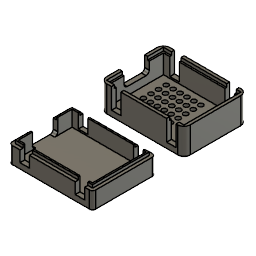
Camera_cover (Autodesk Fusion 360 design; units mm, degrees)
part number: 2026-01-28-19-58-32-867
Autodesk Fusion 360 part; units mm, degrees
note: some values were not read from the file. Chosen so that the rebuilt part matches the saved one: which bodies a step acts on. Set by a fixed rule: which sketch regions a step uses.
sketch "Esquisse1" plane through (0, 0, 0) normal (0, 1, 0) x (1, 0, 0)
  line L0 (23.5, 17) -> (-23.5, 17)
  line L1 (-23.5, 17) -> (-23.5, -17)
  line L2 (-23.5, -17) -> (23.5, -17)
  line L3 (23.5, -17) -> (23.5, 17)
  line L4 (23.5, 17) -> (-23.5, -17) construction
  line L5 (-23.5, 17) -> (23.5, -17) construction
  line L6 (26.5, 20) -> (-26.5, 20)
  line L7 (-26.5, 20) -> (-26.5, -20)
  line L8 (-26.5, -20) -> (26.5, -20)
  line L9 (26.5, -20) -> (26.5, 20)
  line L10 (26.5, 20) -> (-26.5, -20) construction
  line L11 (-26.5, 20) -> (26.5, -20) construction
  dimension "d1" = 47
  dimension "d2" = 34
  dimension "d3" = 40
  dimension "d4" = 53
  constraint horizontal L0
  constraint perpendicular L0 L1
  constraint parallel L0 L2
  constraint parallel L1 L3
  constraint coincident L4 origin
  constraint coincident L5 origin
  constraint horizontal L6
  constraint perpendicular L6 L7
  constraint parallel L6 L8
  constraint parallel L7 L9
  constraint coincident L10 origin
  constraint coincident L11 origin
  measures "d1" distance of L0.start L0.end
  measures "d2" distance of L0.start L2.end
  measures "d3" distance of L6.start L8.end
  measures "d4" distance of L7.end L8.end
extrude "Extrusion1" add sketch "Esquisse1" along normal blind 29 makes body 1
sketch "Esquisse2" plane through (0, 0, 20) normal (0, 0, 1) x (1, 0, 0)
  line L0 (-26.5, 0) -> (26.5, 0)
  line L1 (26.5, 0) -> (26.5, 29)
  line L2 (26.5, 29) -> (-26.5, 29)
  line L3 (-26.5, 29) -> (-26.5, 0)
  line L4 (-26.5, 18) -> (26.5, 18)
  line L5 (26.5, 18) -> (26.5, 17)
  line L6 (26.5, 17) -> (-26.5, 17)
  line L7 (-26.5, 17) -> (-26.5, 18)
  dimension "d8" = 53
  dimension "d9" = 1
  dimension "d10" = 11
  constraint horizontal L4
  constraint vertical L5
  constraint horizontal L6
  constraint vertical L7
  constraint coincident L3 L4.start
  measures "d8" distance of L4.start L4.end
  measures "d9" distance of L4.end L5.end
  measures "d10" distance of L2 L4
extrude "Extrusion2" add sketch "Esquisse1" along normal blind 3 contours L0 L1 L2 L3 bodies 1
extrude "Extrusion3" add sketch "Esquisse1" along normal blind 3 from surface at 26 contours L0 L1 L2 L3 bodies 1
extrude "Extrusion4" cut sketch "Esquisse2" against normal blind 45 contours L1 L3 L4 L5 L6 L7 bodies 1 makes body 2 at (-8.8333, 29, 6.6667)
sketch "Esquisse3" plane through (0, 17, 0) normal (0, 1, 0) x (-1, 0, 0)
  line L0 (-26.5, -20) -> (26.5, -20)
  line L1 (26.5, -20) -> (26.5, 20)
  line L2 (26.5, 20) -> (-26.5, 20)
  line L3 (23.5, -17) -> (-23.5, -17)
  line L4 (-23.5, 17) -> (23.5, 17)
  line L5 (23.5, 17) -> (23.5, -17)
  line L6 (-24.6, -18.1) -> (24.6, -18.1)
  line L7 (24.6, -18.1) -> (24.6, 18.1)
  line L8 (24.6, 18.1) -> (-24.6, 18.1)
  line L9 (-24.6, 18.1) -> (-24.6, -18.1)
  line L10 (-24.6, -18.1) -> (24.6, 18.1) construction
  line L11 (24.6, -18.1) -> (-24.6, 18.1) construction
  line L12 (-26.5, 20) -> (-26.5, -20)
  line L13 (-23.5, -17) -> (-23.5, 17)
  dimension "d18" = 1.1
  dimension "d19" = 1.1
  constraint horizontal L6
  constraint perpendicular L6 L7
  constraint parallel L6 L8
  constraint parallel L7 L9
  constraint coincident L10 origin
  constraint coincident L11 origin
  measures "d18" distance of L3 L6
  measures "d19" distance of L5 L7
extrude "Extrusion5" cut sketch "Esquisse3" against normal blind 2 contours L6 L7 L8 L9 bodies 1
sketch "Esquisse4" plane through (0, 18, 0) normal (0, -1, 0) x (1, 0, 0)
  line L0 (-26.5, -20) -> (26.5, -20)
  line L1 (26.5, 20) -> (-26.5, 20)
  line L2 (-26.5, 20) -> (-26.5, -20)
  line L3 (23.5, -17) -> (-23.5, -17)
  line L4 (-23.5, -17) -> (-23.5, 17)
  line L5 (-23.5, 17) -> (23.5, 17)
  line L6 (21.9, 15.4) -> (-21.9, -15.4) construction
  line L7 (-21.9, 15.4) -> (21.9, -15.4) construction
  line L8 (-24.5, 18) -> (24.5, 18)
  line L9 (24.5, 18) -> (24.5, -18)
  line L10 (24.5, -18) -> (-24.5, -18)
  line L11 (-24.5, -18) -> (-24.5, 18)
  line L12 (-24.5, 18) -> (24.5, -18) construction
  line L13 (24.5, 18) -> (-24.5, -18) construction
  line L14 (26.5, -20) -> (26.5, 20)
  line L15 (23.5, 17) -> (23.5, -17)
  dimension "d51" = 1
  dimension "d74" = 1
  constraint coincident L6 origin
  constraint coincident L7 origin
  constraint horizontal L8
  constraint perpendicular L8 L9
  constraint parallel L8 L10
  constraint parallel L9 L11
  constraint coincident L12 origin
  constraint coincident L13 origin
  measures "d51" distance of L5 L8
  measures "d74" distance of L9 L15
extrude "Extrusion6" add sketch "Esquisse4" along normal blind 1.9 contours L8 L9 L10 L11 bodies 2
fillet "Congé1" radius 2 4 edges at (26.5, 23.5, -20) (26.5, 23.5, 20) (-26.5, 23.5, 20) (-26.5, 23.5, -20) on bodies 2
fillet "Congé2" radius 4 2 edges at (-26.5, 8.5, -20) (-26.5, 8.5, 20) on bodies 1
fillet "Congé2" radius 4 2 edges at (26.5, 8.5, -20) (26.5, 8.5, 20) on bodies 1
sketch "Esquisse5" plane through (0, 0, 20) normal (0, 0, 1) x (1, 0, 0)
  line L0 (-24.5, 29) -> (-24.5, 18)
  line L1 (-24.5, 18) -> (24.5, 18)
  line L2 (24.5, 18) -> (24.5, 29)
  line L3 (24.5, 29) -> (-24.5, 29)
  line L4 (-19.5, 4) -> (-13.5, 4)
  line L5 (-13.5, 4) -> (-13.5, 25)
  line L6 (-13.5, 25) -> (-19.5, 25)
  line L7 (-19.5, 25) -> (-19.5, 4)
  line L8 (-22.5, 0) -> (-22.5, 17)
  line L9 (-22.5, 0) -> (22.5, 0)
  line L10 (21.5, 4) -> (15.5, 4)
  line L11 (15.5, 4) -> (15.5, 25)
  line L12 (15.5, 25) -> (21.5, 25)
  line L13 (21.5, 25) -> (21.5, 4)
  dimension "d30" = 3
  dimension "d31" = 4
  dimension "d32" = 4
  dimension "d34" = 4
  dimension "d35" = 4
  dimension "d71" = 3
  dimension "d72" = 6
  dimension "d73" = 6
  constraint horizontal L4
  constraint vertical L5
  constraint horizontal L6
  constraint vertical L7
  constraint horizontal L10
  constraint vertical L11
  constraint horizontal L12
  constraint vertical L13
  measures "d30" distance of L7 L8
  measures "d31" distance of L4 L9
  measures "d32" distance of L3 L6
  measures "d34" distance of L9 L10
  measures "d35" distance of L3 L12
  measures "d71" distance of L2 L13
  measures "d72" distance of L11 L13
  measures "d73" distance of L5 L7
extrude "Extrusion7" cut sketch "Esquisse5" against normal blind 94 contours L1 L5 L6 L7 | L1 L4 L5 L7 | L1 L10 L11 L13 | L1 L11 L12 L13 bodies 1 2
sketch "Esquisse6" plane through (0, 0, 0) normal (0, -1, 0) x (1, 0, 0)
  line L0 (26.5, -16) -> (26.5, 16)
  line L1 (22.5, 20) -> (-22.5, 20)
  arc A0 (-22.5, 20) -> (-26.5, 16) centre (-22.5, 16) ccw
  line L2 (-26.5, 16) -> (-26.5, -16)
  arc A1 (-26.5, -16) -> (-22.5, -20) centre (-22.5, -16) ccw
  line L3 (-22.5, -20) -> (22.5, -20)
  circle A2 centre (17, 3) radius 4.5
  arc A3 (26.5, 16) -> (22.5, 20) centre (22.5, 16) ccw
  arc A4 (22.5, -20) -> (26.5, -16) centre (22.5, -16) ccw
  dimension "d38" = 9
  dimension "d39" = 17
  dimension "d41" = 9.5
  measures "d38" diameter of A2
  measures "d39" distance of L1 A2.centre
  measures "d41" distance of L0 A2.centre
hole "Perçage1" at (5.0138, 0, -12.1907) direction (0, 1, 0) diameter 3 depth 13 tip angle 118 bodies 1
pattern_linear "Réseau R1" count 6 spacing 4.8 along (0, 0, 1) count 6 spacing 4.4 along (-1, 0, 0) of "Perçage1"
extrude "Extrusion8" cut sketch "Esquisse6" against normal blind 15 contours A2 bodies 1
sketch "Esquisse7" plane through (-26.5, 0, 0) normal (-1, 0, 0) x (0, 0, 1)
  line L0 (16, 0) -> (16, 17)
  line L1 (16, 17) -> (-16, 17)
  line L2 (-16, 17) -> (-16, 0)
  line L3 (-16, 0) -> (16, 0)
  line L4 (8, 8) -> (-8, 8)
  line L5 (-8, 8) -> (-8, 26)
  line L6 (-8, 26) -> (8, 26)
  line L7 (8, 26) -> (8, 8)
  line L8 (-18, 29) -> (18, 29)
  dimension "d65" = 8
  dimension "d66" = 3
  dimension "d67" = 8
  dimension "d68" = 8
  constraint horizontal L4
  constraint vertical L5
  constraint horizontal L6
  constraint vertical L7
  measures "d65" distance of L3 L4
  measures "d66" distance of L6 L8
  measures "d67" distance of L2 L5
  measures "d68" distance of L0 L7
extrude "Extrusion12" cut sketch "Esquisse7" against normal blind 4 contours L1 L4 L5 L7 | L1 L5 L6 L7 bodies 1 2
fillet "Congé4" radius 2 4 edges at (-25, 8, -8) (-25, 8, 8) (-25, 26, 8) (-25, 26, -8) on bodies 1 2
move_body "Déplacer1" bodies 2 to x (1, 0, 0) y (0, -1, 0) z (0, 0, -1) at (0, 29.2, 43)
move_body "Déplacer2" bodies 1 to x (1, 0, 0) y (0, 1, 0) z (0, 0, 1) at (0, 0, -15)
fillet "Congé5" radius 0.5 16 edges at (-26.5, 0, -15) (-25.3284, 0, 3.8284) (0, 0, 5) (25.3284, 0, 3.8284) (26.5, 0, -15) (25.3284, 0, -33.8284) (0, 0, -35) (-25.3284, 0, -33.8284) (25.9142, 0.2, 23.5858) (26.5, 0.2, 43) (25.9142, 0.2, 62.4142) (0, 0.2, 63) (-25.9142, 0.2, 62.4142) (-26.5, 0.2, 43) (-25.9142, 0.2, 23.5858) (0, 0.2, 23) on bodies 1 2
equation "d4 = 47 mm + 6 mm"
equation "d41 = 4.5 mm + 5 mm"
